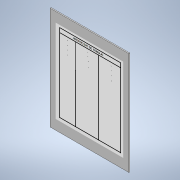
# Autodesk Inventor part: Tabla_Instructivo
Saved by Autodesk Inventor 2021 (Build 250183000, 183)
## iProperties
Created: 2021-07-11
Part Number: Tabla_Instructivo
Material: Generic
Document SubType Name: Modeling
Designer: Nelson
Density: 1 g/cm^3
Appearance: Default
Author: Nelson
Autodesk Inventor part; units mm, degrees
ref_plane "YZ Plane" through (0, 0, 0) normal (1, 0, 0) x (0, 1, 0)
ref_plane "XZ Plane" through (0, 0, 0) normal (0, 1, 0) x (-1, 0, 0)
ref_plane "XY Plane" through (0, 0, 0) normal (0, 0, 1) x (1, 0, 0)
sketch "Sketch1" plane through (0, 0, 0) normal (0, 0, 1) x (1, 0, 0)
  line L0 (0, 0) -> (230, 0)
  line L1 (230, 0) -> (230, 300)
  line L2 (230, 300) -> (0, 300)
  line L3 (0, 300) -> (0, 0)
  dimension "d0" = 300
  dimension "d1" = 230
  constraints: 8 end point, 2 parallel, 1 horizontal, 1 perpendicular
  measures "d0" distance of L0.end L1.end
  measures "d1" distance of L1.end L2.end
extrude "Extrusion1" add sketch "Sketch1" along normal blind 3
sketch "Sketch2" plane through (0, 0, 3) normal (0, 0, 1) x (1, 0, 0)
  line L0 (16.72, 271.67) -> (213.279, 271.67) construction
  line L1 (213.279, 271.67) -> (213.279, 28.33) construction
  line L2 (213.279, 28.33) -> (16.72, 28.33) construction
  line L3 (16.72, 28.33) -> (16.72, 271.67) construction
  line L4 (0, 300) -> (0, 0) projected
  line L5 (0, 0) -> (230, 0) projected
  line L6 (230, 300) -> (0, 300) projected
  dimension "d24" = 16.72
  dimension "d27" = 28.33
  dimension "d30" = 28.33
  constraints: 2 other
  measures "d24" distance between parallel lines of L3 L4
  measures "d27" distance between parallel lines of L5 L2
  measures "d30" distance between parallel lines of L6 L0
decal "Decal1"
body "Solid1"
